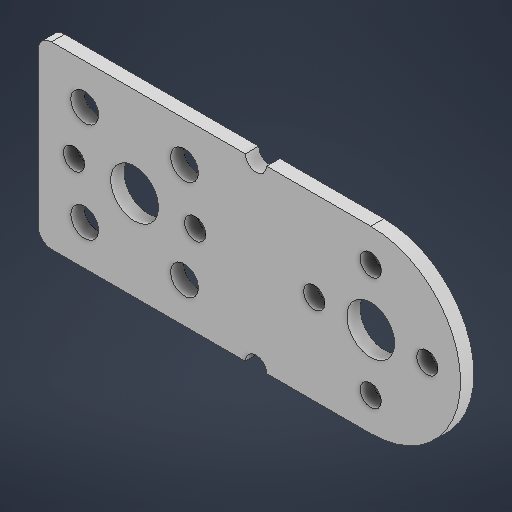
# Autodesk Inventor part: motor holder bracket
Saved by Autodesk Inventor 2027.1 (Build 311270010, 270A)
## iProperties
Created: 2026-05-03
Part Number: motor holder bracket
Material: Generic
Document SubType Name: Modeling
Designer: ganak
Density: 1 g/cm^3
Appearance: Default
Author: ganak
Autodesk Inventor part; units mm, degrees
ref_plane "YZ Plane" through (0, 0, 0) normal (1, 0, 0) x (0, 1, 0)
ref_plane "XZ Plane" through (0, 0, 0) normal (0, 1, 0) x (-1, 0, 0)
ref_plane "XY Plane" through (0, 0, 0) normal (0, 0, 1) x (1, 0, 0)
sketch "Sketch1" plane through (0, 0, 0) normal (0, 0, 1) x (1, 0, 0)
  line L0 (2, 0) -> (63.5, 0)
  line L1 (63.5, 0) -> (63.5, 27) construction
  line L2 (63.5, 27) -> (2, 27)
  line L3 (0, 25) -> (0, 2)
  circle A0 centre (50, 13.5) radius 13.5
  circle A1 centre (50, 13.5) radius 3.6
  circle A2 centre (58.5, 13.5) radius 1.6
  circle A3 centre (50, 13.5) radius 8.5 construction
  line L4 (50, 13.5) -> (58.5, 13.5) construction
  circle A4 centre (50, 22) radius 1.6
  circle A5 centre (41.5, 13.5) radius 1.6
  circle A6 centre (50, 5) radius 1.6
  circle A7 centre (14.5, 13.5) radius 3.6
  line L5 (7, 21) -> (22, 21) construction
  line L6 (22, 21) -> (22, 6) construction
  line L7 (22, 6) -> (7, 6) construction
  line L8 (7, 6) -> (7, 21) construction
  line L9 (7, 21) -> (22, 6) construction
  line L10 (22, 21) -> (7, 6) construction
  circle A8 centre (7, 21) radius 2.1
  circle A9 centre (7, 6) radius 2.1
  circle A10 centre (22, 6) radius 2.1
  circle A11 centre (22, 21) radius 2.1
  arc A12 (2, 27) -> (0, 25) centre (2, 25) ccw
  arc A13 (0, 2) -> (2, 0) centre (2, 2) ccw
  circle A14 centre (5.4, 13.5) radius 1.6
  circle A15 centre (23.6, 13.5) radius 1.6
  circle A16 centre (32.75, 27) radius 1.6
  circle A17 centre (32.75, 0) radius 1.6
  point P0 (0, 0)
  point P1 (0, 27)
  point P2 (50, 0)
  point P3 (50, 27)
  point P4 (34.35, 27)
  point P5 (31.15, 27)
  point P6 (31.15, 0)
  point P7 (34.35, 0)
  dimension "d5" = 17
  dimension "d2" = 13.5
  dimension "d3" = 7.2
  dimension "d4" = 50
  dimension "d6" = 3.2
  dimension "d9" = 360
  dimension "d11" = 4.2
  dimension "d12" = 2
  dimension "d13" = 7
  dimension "d14" = 15
  constraints: 22 end point, 17 centre point, 9 equal radius, 9 tangent, 7 point on line, 6 coincident, 4 midpoint, 4 parallel, 4 point on circle, 3 horizontal, 3 perpendicular, 1 horizontal alignment, 11 other
  measures "d2" distance from line of L1 A0.centre
  measures "d3" diameter of A1
  measures "d4" distance from line of L3 A0.centre
  measures "d6" diameter of A2
  measures "d11" diameter of A11
  measures "d12" radius of A12
  measures "d13" distance between parallel lines of L3 L8
  measures "d14" distance of L5.start L5.end
extrude "Extrusion1" add sketch "Sketch1" along normal blind 2 contours A13 L3 A12 L2 A16 A0 L0 A17 | A0
body "Solid1"
